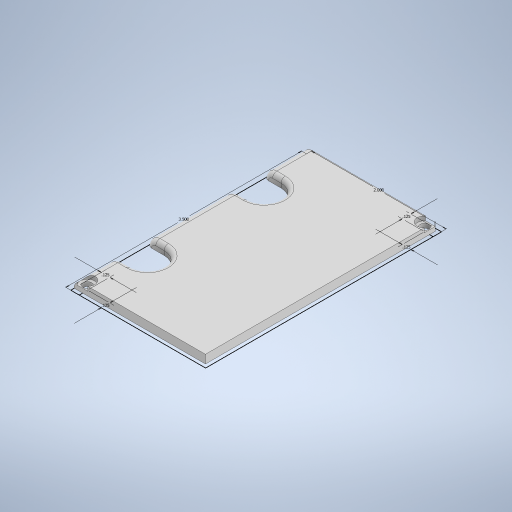
# Autodesk Inventor part: AFL-102-001-02-2A DualSensorReadout - Lid - w front homes
Saved by Autodesk Inventor 2024.1 (Build 281209000, 209)
## iProperties
Created: 2024-01-28
Part Number: AFL-102-001-02-2A DualSensorReadout - Lid - w front homes
Material: Generic
Document SubType Name: Modeling
Designer: Beaucage
Density: 1 g/cm^3
Appearance: Default
Author: Beaucage
Autodesk Inventor part; units mm, degrees
ref_plane "YZ Plane" through (0, 0, 0) normal (1, 0, 0) x (0, 1, 0)
ref_plane "XZ Plane" through (0, 0, 0) normal (0, 1, 0) x (-1, 0, 0)
ref_plane "XY Plane" through (0, 0, 0) normal (0, 0, 1) x (1, 0, 0)
sketch "Sketch1" plane through (0, 0, 0) normal (0, 1, 0) x (-1, 0, 0)
  line L0 (0, 0) -> (50.8, 0)
  line L1 (50.8, 0) -> (50.8, -88.9)
  line L2 (50.8, -88.9) -> (0, -88.9)
  line L3 (0, -88.9) -> (0, 0)
  line L4 (50.8, 0) -> (47.625, 0)
  line L5 (47.625, 0) -> (47.625, -3.175)
  line L6 (47.625, -3.175) -> (50.8, -3.175)
  line L7 (50.8, -3.175) -> (50.8, 0)
  line L8 (0, -88.9) -> (3.175, -88.9)
  line L9 (3.175, -88.9) -> (3.175, -85.725)
  line L10 (3.175, -85.725) -> (0, -85.725)
  line L11 (0, -85.725) -> (0, -88.9)
  dimension "d0" = 50.8
  dimension "d1" = 88.9
  dimension "d2" = 3.175
  dimension "d3" = 3.175
  dimension "d4" = 3.175
  dimension "d5" = 3.175
  constraints: 24 end point, 6 parallel, 3 horizontal, 3 perpendicular
  measures "d0" distance of L1.end L2.end
  measures "d1" distance of L0.end L1.end
  measures "d2" distance of L6.end L5.end
  measures "d3" distance of L5.end L4.end
  measures "d4" distance of L10.end L9.end
  measures "d5" distance of L9.end L8.end
extrude "Extrusion1" add sketch "Sketch1" along normal blind 3.175
sketch "Sketch2" plane through (0, 3.175, 0) normal (0, 1, 0) x (1, 0, 0)
  line L0 (-50.8, 0) -> (0, 0) projected
  line L1 (-50.8, 0) -> (-47.625, 0)
  line L2 (-47.625, 0) -> (-47.625, 3.175)
  line L3 (-47.625, 3.175) -> (-50.8, 3.175)
  line L4 (-50.8, 3.175) -> (-50.8, 0)
  line L5 (0, 88.9) -> (-50.8, 88.9) projected
  line L6 (0, 88.9) -> (-3.175, 88.9)
  line L7 (-3.175, 88.9) -> (-3.175, 85.725)
  line L8 (-3.175, 85.725) -> (0, 85.725)
  line L9 (0, 85.725) -> (0, 88.9)
  dimension "d15" = 3.175
  dimension "d16" = 3.175
  dimension "d17" = 3.175
  dimension "d18" = 3.175
  constraints: 16 end point, 4 parallel, 2 horizontal, 2 perpendicular
  measures "d15" distance of L3.end L2.end
  measures "d16" distance of L2.end L1.end
  measures "d17" distance of L8.end L7.end
  measures "d18" distance of L7.end L6.end
hole "Hole2" at (-47.625, 3.175, -3.175) at (-3.175, 3.175, -85.725) direction (0, -1, 0) diameter 3.2766 depth 7.9375 counterbore diameter 5.5626 counterbore depth 1.5875 clearance for "Socket Head Cap Screw" size "#4" standard "Ansi Unified Screw Threads"
fillet "Fillet1" radius 3.175 1 edges at (-50.8, 3.175, -44.45)
sketch "Sketch3" plane through (0, 3.175, 0) normal (0, 1, 0) x (1, 0, 0)
  line L0 (-50.8, 88.9) -> (-50.8, 0) projected
  line L1 (0, 89.1361) -> (-50.8, 89.1361)
  line L2 (-50.8, 89.1361) -> (-50.8, 87.8661)
  line L3 (-50.8, 87.8661) -> (0, 87.8661)
  line L4 (0, 87.8661) -> (0, 89.1361)
  line L5 (-47.625, 0) -> (0, 0) projected
  line L6 (0, 89.1361) -> (-1.27, 89.1361)
  line L7 (-1.27, 89.1361) -> (-1.27, 0)
  line L8 (-1.27, 0) -> (0, 0)
  line L9 (0, 0) -> (0, 89.1361)
  line L10 (0, 0) -> (-50.8, 0)
  line L11 (-50.8, 0) -> (-50.8, 1.27)
  line L12 (-50.8, 1.27) -> (0, 1.27)
  line L13 (0, 1.27) -> (0, 0)
  line L14 (-50.8, 89.1361) -> (-50.8, 66.5809)
  line L15 (-50.8, 0) -> (-50.8, 22.5552)
  line L16 (-50.8, 22.5552) -> (-44.45, 22.5552)
  circle A0 centre (-44.45, 22.5552) radius 5.08
  line L17 (-47.625, 5.9563) -> (-47.625, 88.9) projected
  line L18 (-50.8, 66.5809) -> (-44.45, 66.5809) construction
  line L19 (-50.8, 60.2309) -> (-44.45, 60.2309)
  line L20 (-44.45, 72.9309) -> (-50.8, 72.9309)
  arc A1 (-50.8, 72.9309) -> (-50.8, 60.2309) centre (-50.8, 66.5809) ccw
  arc A2 (-44.45, 60.2309) -> (-44.45, 72.9309) centre (-44.45, 66.5809) ccw
  line L21 (-50.8, 22.5552) -> (-44.45, 22.5552) construction
  line L22 (-50.8, 16.2052) -> (-44.45, 16.2052)
  line L23 (-44.45, 28.9052) -> (-50.8, 28.9052)
  arc A3 (-50.8, 28.9052) -> (-50.8, 16.2052) centre (-50.8, 22.5552) ccw
  arc A4 (-44.45, 16.2052) -> (-44.45, 28.9052) centre (-44.45, 22.5552) ccw
  line L24 (-47.625, 28.9052) -> (-50.8, 28.9052)
  point P0 (-1.27, 1.27)
  point P1 (-1.27, 87.8661)
  point P2 (-47.625, 66.5809)
  point P3 (-47.625, 22.5552)
  point P4 (-47.625, 26.5208)
  point P5 (-49.53, 22.5552)
  dimension "d27" = 1.27
  dimension "d28" = 1.27
  dimension "d29" = 1.27
  dimension "d30" = 22.5552
  dimension "d31" = 22.5552
  dimension "d32" = 6.35
  dimension "d33" = 10.16
  dimension "d40" = 12.7
  dimension "d41" = 12.7
  constraints: 48 end point, 9 tangent, 8 parallel, 8 point on circle, 6 perpendicular, 5 centre point, 5 point on line, 3 horizontal, 3 midpoint, 1 coincident, 1 collinear, 1 other
  measures "d27" distance of L2.end L1.end
  measures "d28" distance of L8.end L7.end
  measures "d29" distance of L10.end L11.end
  measures "d30" distance of L1.end L14.end
  measures "d31" distance of L10.end L15.end
  measures "d32" distance of L15.end L16.end
  measures "d33" diameter of A0
  measures "d40" diameter of A2
  measures "d41" diameter of A4
extrude "Extrusion2" cut sketch "Sketch3" against normal through all contours L2 L1 L7 L3 L0 | L20 L17 L19 L0 | L1 L4 L3 L7 | L20 A2 L19 L17 | L3 L9 L12 L7 | L23 L17 A0 L16 L0 | L0 A3 | L12 L9 L5 L7 | L7 L5 L10 L0 L12 | L23 A4 L22 L17 A0 | L16 A0 L17 L22 L0 | L17 L16 A0 | A0 L17 | L16 L17 A0
fillet "Fillet2" radius 1.5875 10 edges at (-46.0375, 3.175, -16.2052) (-49.8701, 2.2451, -16.2052) (-46.0375, 3.175, -28.9052) (-49.8701, 2.2451, -28.9052) (-38.1, 3.175, -22.5552) (-46.0375, 3.175, -60.2309) (-49.8701, 2.2451, -60.2309) (-46.0375, 3.175, -72.9309) (-49.8701, 2.2451, -72.9309) (-38.1, 3.175, -66.5809)
body "Solid1"
